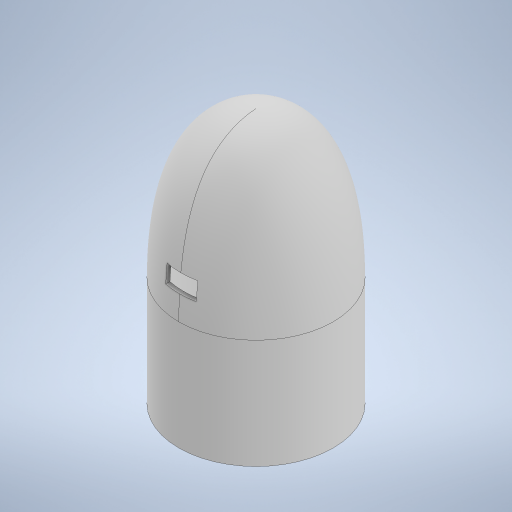
# Autodesk Inventor part: Cone
Saved by Autodesk Inventor 2023.2 (Build 272271030, 271C)
## iProperties
Created: 2023-02-11
Part Number: Cone
Material: Generic
Document SubType Name: Modeling
Designer: Lukas
Density: 1 g/cm^3
Appearance: Default
polomer: 33.200 mm
drazka: 50.000 mm
vyska: 200.000 mm
tloustka: 2.000 mm
pcb: 66.000 mm
d26: 1.500 mm
d27: 75.000 mm
Author: Lukas
Autodesk Inventor part; units mm, degrees
ref_plane "YZ Plane" through (0, 0, 0) normal (1, 0, 0) x (0, 1, 0)
ref_plane "XZ Plane" through (0, 0, 0) normal (0, 1, 0) x (-1, 0, 0)
ref_plane "XY Plane" through (0, 0, 0) normal (0, 0, 1) x (1, 0, 0)
sketch "Cone Sketch" plane through (0, 0, 0) normal (1, 0, 0) x (0, 1, 0)
  line L0 (8.1025, 33.3) -> (72.3676, 33.8) construction
  line L1 (72.3676, 33.8) -> (73.4955, 0) construction
  spline S0 degree 2 poles (8.1025, 33.3) (72.3676, 33.8) (73.4955, 0) knots 1 1 1 2 2 2
  line L2 (8.1025, 35.3) -> (72.2508, 35.3) construction
  line L3 (72.2508, 35.3) -> (75, 0) construction
  spline S1 degree 2 poles (8.1025, 35.3) (72.2508, 35.3) (75, 0) knots 1 1 1 2 2 2
  line L4 (75, 0) -> (73.4955, 0)
  line L5 (75, 0) -> (0, 0)
  line L6 (8.1025, 35.3) -> (-41.8975, 35.3)
  line L7 (-41.8975, 35.3) -> (-41.8975, 34.3)
  line L8 (-41.8975, 34.3) -> (8.1025, 34.3)
  line L9 (8.1025, 34.3) -> (8.1025, 33.3)
  line L10 (-79.1738, 0) -> (181.7601, 0) projected
  point P0 (8.1025, 33.8)
  point P1 (-41.8975, 34.8)
  point P2 (144.4838, 14.0682)
  point P3 (31.2287, 39.0196)
  dimension "d26" = 1.5
  dimension "d27" = 75
  dimension "d61" = 1
  dimension "d63" = 50
  dimension "d70" = 34.3
  constraints: 12 end point, 5 horizontal, 3 perpendicular, 2 midpoint, 2 parallel, 1 horizontal alignment, 1 point on line, 6 other
  measures "d26" distance from line of L1.end L3
  measures "d27" distance of L5.end L3.end
  measures "d61" distance between parallel lines of L6 L8
  measures "d63" horizontal distance of point (8.102, 33.8) point (-41.898, 34.8)
  measures "d70" distance between parallel lines of L8 L5
revolve "Cone" add sketch "Cone Sketch" angle 360 about axis through (0, -10, 0) along (0, 1, 0)
sketch "Sketch2" plane through (0, 0, 0) normal (0, 0, 1) x (1, 0, 0)
  line L0 (3, -20.8975) -> (-3, -20.8975)
  line L1 (-3, -20.8975) -> (-3, -26.8975)
  line L2 (-3, -26.8975) -> (3, -26.8975)
  line L3 (3, -26.8975) -> (3, -20.8975)
  line L4 (35.3, 8.1025) -> (-35.3, 8.1025) projected
  point P0 (0, 0)
  point P1 (-3, -23.8975)
  point P2 (0, 8.1025)
  dimension "d71" = 3
  dimension "d72" = 6
  dimension "d73" = 6
  dimension "d77" = 29
  constraints: 8 end point, 2 parallel, 1 horizontal, 1 midpoint, 1 perpendicular
  measures "d71" distance from line of L1 point (0, 0)
  measures "d72" distance from line of point (-3, -23.898) L3
  measures "d73" distance between parallel lines of L2 L0
  measures "d77" distance between parallel lines of L0 L4
extrude "RBF+ Breakout  Hole" [suppressed]
sketch "Sketch4" plane through (0, 0, 0) normal (0, 0, 1) x (1, 0, 0)
  line L0 (7, 27.102) -> (-7, 27.102)
  line L1 (-7, 27.102) -> (-7, 19.102)
  line L2 (-7, 19.102) -> (7, 19.102)
  line L3 (7, 19.102) -> (7, 27.102)
  line L4 (-11.9, 0) -> (11.9, 0) projected
  line L5 (0, -5.6204) -> (0, 33.7224) projected
  point P0 (0, 0)
  point P1 (-7, 23.102)
  dimension "d78" = 19.102
  dimension "d79" = 8
  dimension "d80" = 7
  dimension "d81" = 7
  constraints: 8 end point, 2 parallel, 1 horizontal, 1 midpoint, 1 perpendicular
  measures "d78" distance between parallel lines of L4 L2
  measures "d79" distance between parallel lines of L2 L0
  measures "d80" distance from line of point (-7, 23.102) L5
  measures "d81" distance between parallel lines of L3 L5
extrude "Extrusion2" cut sketch "Sketch4" along normal mid plane 100
equation "\"d72\" = 2 * d71"
equation "\"d73\" = 2 * d71"
equation "\"gap\" = 0.1"
equation "\"sdcard_offset\" = 15"
body "Solid4"
